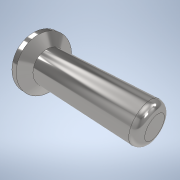
# Autodesk Inventor part: Гвоздик 3 мм
Saved by Autodesk Inventor 2021.1 (Build 251245010, 245A)
## iProperties
Created: 2026-05-06
Part Number: Гвоздик 3 мм
Material: Типовые
Document SubType Name: Modeling
Designer: Андрей Тарасов
Density: 1 g/cm^3
Appearance: По умолчанию
Author: Андрей Тарасов
Autodesk Inventor part; units mm, degrees
ref_plane "YZ Plane" through (0, 0, 0) normal (1, 0, 0) x (0, 1, 0)
ref_plane "XZ Plane" through (0, 0, 0) normal (0, 1, 0) x (-1, 0, 0)
ref_plane "XY Plane" through (0, 0, 0) normal (0, 0, 1) x (1, 0, 0)
sketch "Эскиз3" plane through (0, 0, 0) normal (0, 0, 1) x (1, 0, 0)
  line L0 (0, 0) -> (0, 2.5)
  line L1 (0, 2.5) -> (0.5, 2.5)
  line L2 (0.5, 2.5) -> (1, 1.5)
  line L3 (1, 1.5) -> (9.4, 1.5)
  line L4 (10, 0.9) -> (10, 0)
  line L5 (10, 0) -> (0, 0)
  arc A0 (10, 0.9) -> (9.4, 1.5) centre (9.4, 0.9) ccw
  point P0 (10, 1.5)
  dimension "d9" = 2.5
  dimension "d10" = 0.5
  dimension "d11" = 1.5
  dimension "d12" = 1
  dimension "d13" = 10
  dimension "d15" = 0.6
  constraints: 12 end point, 3 perpendicular, 2 point on circle, 2 point on line, 2 tangent, 1 centre point, 1 vertical
  measures "d9" distance of L0.start L0.end
  measures "d10" distance of L0.end L1.end
  measures "d11" distance of point (10, 1.5) L4.end
  measures "d12" distance from line of L0 L2.end
  measures "d13" distance between parallel lines of L0 L4
  measures "d15" radius of A0
revolve "Вращение1" add sketch "Эскиз3" angle 360 about axis through (10, 0, 0) along (-1, 0, 0)
